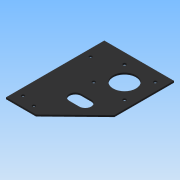
# Autodesk Inventor part: пластина  экструдера
Saved by Autodesk Inventor 2017 (Build 210142000, 142)
## iProperties
Part Number: пластина  экструдера
Material: Типовые
Document SubType Name: Modeling
Designer: Max
Mass: 9.01175 g
Surface Area: 117.642 cm^2
Volume: 9.01175 cm^3
Density: 1 g/cm^3
Appearance: Резина — черная
Author: Max
Autodesk Inventor part; units mm, degrees
ref_plane "YZ Plane" through (0, 0, 0) normal (1, 0, 0) x (0, 1, 0)
ref_plane "XZ Plane" through (0, 0, 0) normal (0, 1, 0) x (-1, 0, 0)
ref_plane "XY Plane" through (0, 0, 0) normal (0, 0, 1) x (1, 0, 0)
sketch "Эскиз1" plane through (0, 0, 0) normal (0, 0, 1) x (1, 0, 0)
  line L0 (15.5, 15.5) -> (-15.5, 15.5) construction
  line L1 (-15.5, 15.5) -> (-15.5, -15.5) construction
  line L2 (-15.5, -15.5) -> (15.5, -15.5) construction
  line L3 (15.5, -15.5) -> (15.5, 15.5) construction
  line L4 (15.5, 15.5) -> (-15.5, -15.5) construction
  line L5 (-15.5, 15.5) -> (15.5, -15.5) construction
  circle A0 centre (-15.5, 15.5) radius 1.6
  circle A1 centre (15.5, 15.5) radius 1.6
  circle A2 centre (15.5, -15.5) radius 1.6
  circle A3 centre (-15.5, -15.5) radius 1.6
  circle A4 centre (0, 0) radius 11.5
  line L6 (-46.3, 25.9) -> (23.9, 25.9)
  line L7 (23.9, 25.9) -> (23.9, -34.1)
  line L8 (-16.1, -73.1) -> (-46.3, -73.1)
  line L9 (-46.3, -73.1) -> (-46.3, 25.9)
  line L10 (-16.1, -73.1) -> (23.9, -34.1)
  line L11 (-11.3, -38.3) -> (-1.3, -38.3) construction
  line L12 (-11.3, -32.3) -> (-1.3, -32.3)
  line L13 (-1.3, -44.3) -> (-11.3, -44.3)
  arc A5 (-11.3, -32.3) -> (-11.3, -44.3) centre (-11.3, -38.3) ccw
  arc A6 (-1.3, -44.3) -> (-1.3, -32.3) centre (-1.3, -38.3) ccw
  circle A7 centre (-39.1, 14.9) radius 1.5
  circle A8 centre (-39.1, -52.1) radius 1.5
  circle A9 centre (-24.8, -66.5) radius 1.5
  point P0 (-6.3, -38.3)
  dimension "d0" = 31
  dimension "d1" = 31
  dimension "d2" = 3.2
  dimension "d3" = 3.2
  dimension "d4" = 3.2
  dimension "d5" = 3.2
  dimension "d6" = 23
  dimension "d7" = 6.8
  dimension "d8" = 8.4
  dimension "d9" = 8.8
  dimension "d10" = 70.2
  dimension "d11" = 60
  dimension "d12" = 99
  dimension "d13" = 40
  dimension "d14" = 22
  dimension "d15" = 12
  dimension "d16" = 20.8
  dimension "d17" = 29
  dimension "d18" = 3
  dimension "d19" = 3
  dimension "d20" = 7.2
  dimension "d21" = 7.2
  dimension "d22" = 67
  dimension "d23" = 21
  dimension "d24" = 58.2
  dimension "d25" = 3
  dimension "d26" = 21.5
  dimension "d27" = 6.6
  constraints: 30 end point, 10 centre point, 5 coincident, 5 parallel, 4 point on circle, 4 tangent, 3 horizontal, 3 midpoint, 2 perpendicular
  measures "d0" distance of L2.end L1.end
  measures "d1" distance of L1.end L0.end
  measures "d2" diameter of A0
  measures "d3" diameter of A1
  measures "d4" diameter of A2
  measures "d5" diameter of A3
  measures "d6" diameter of A4
  measures "d7" distance edge to line of A2 L7
  measures "d8" distance from line of L7 L2.end
  measures "d9" distance edge to line of A1 L6
  measures "d10" distance between parallel lines of L7 L9
  measures "d11" distance of L6.end L7.end
  measures "d12" distance between parallel lines of L6 L8
  measures "d13" horizontal distance of L8.start L7.end
  measures "d15" distance between parallel lines of L13 L12
  measures "d16" distance edge to line of A4 L12
  measures "d17" distance edge to line of A5 L9
  measures "d18" diameter of A7
  measures "d19" diameter of A8
  measures "d20" distance from line of L9 A7.centre
  measures "d21" distance from line of L9 A8.centre
  measures "d22" distance of A8.centre A7.centre
  measures "d23" distance from line of A8.centre L8
  measures "d24" distance between parallel lines of L12 L6
  measures "d25" diameter of A9
  measures "d26" distance from line of A9.centre L9
  measures "d27" distance from line of L8 A9.centre
extrude "Выдавливание1" add sketch "Эскиз1" along normal blind 1.65
fillet "Сопряжение1" radius 3 5 edges at (23.9, 25.9, 0.825) (-46.3, 25.9, 0.825) (23.9, -34.1, 0.825) (-16.1, -73.1, 0.825) (-46.3, -73.1, 0.825)
